Autodesk Fusion 360 part; units mm, degrees
(part 3 of 3)
extrude "돌출9" cut sketch "스케치1" against normal blind 9.6 contours L19 L20 L21 L22 | L23 L24 L25 L26 | L27 L28 L29 L30 bodies 2 in component "leftBody1"
extrude "돌출7'''" add sketch "스케치2 (6)" against normal blind 12 contours L2 L6 L11 L12 L13 L14 L15 L16 L17 L18 | L2 L6 L19 L20 L21 L22 L23 L24 L25 L26 bodies 9 in component "rightPalmRest1"
extrude "돌출8''" cut sketch "스케치2 (6)" against normal blind 12 contours L2 L6 L11 L12 L13 L14 L15 L16 L17 L18 | L2 L6 L19 L20 L21 L22 L23 L24 L25 L26 bodies 9 in component "rightPalmRest1"
extrude "돌출8'''" cut sketch "스케치2 (6)" against normal blind 12 contours L2 L6 L11 L12 L13 L14 L15 L16 L17 L18 | L2 L6 L19 L20 L21 L22 L23 L24 L25 L26 bodies 11 in component "rightPalmRest2"
move_face "면 간격띄우기3" offset -0.5 16 faces at (127.7167, -70, -11) (125.05, -72.6667, -11) (123.05, -74, -11) (122.05, -66, -11) (124.05, -62, -11) (126.3833, -66, -11) (123.05, -67.3333, -3) (122.05, -22, -11) (124.05, -18, -11) (126.3833, -22, -11) (123.05, -23.3333, -3) (127.7167, -26, -11) (125.05, -28.6667, -11) (123.05, -30, -11) (125.05, -64.6667, -11) (125.05, -20.6667, -11) on bodies 11 in component "rightPalmRest2"
extrude "돌출9'" add sketch "스케치2 (6)" against normal blind 12 contours L2 L6 L11 L12 L13 L14 L15 L16 L17 L18 | L2 L6 L19 L20 L21 L22 L23 L24 L25 L26 bodies 9 in component "rightPalmRest1"
component "leftKey1" placed x (1, 0, 0) y (0, 1, 0) z (0, 0, 1) at (0, 0, 0)
component "leftBody1" placed x (1, 0, 0) y (0, 1, 0) z (0, 0, 1) at (0, 0, 0)
component "rightKey1" placed x (1, 0, 0) y (0, 1, 0) z (0, 0, 1) at (0, 0, 0)
component "rightKey2" placed x (1, 0, 0) y (0, 1, 0) z (0, 0, 1) at (0, 0, 0)
component "rightBody1" placed x (1, 0, 0) y (0, 1, 0) z (0, 0, 1) at (0, 0, 0)
component "rightBody2" placed x (1, 0, 0) y (0, 1, 0) z (0, 0, 1) at (0, 0, 0)
component "tempJoin" placed x (1, 0, 0) y (0, 1, 0) z (0, 0, 1) at (13.5824, 154.2275, -3.4182)
component "rightPalmRest1" placed x (1, 0, 0) y (0, 1, 0) z (0, 0, 1) at (0, 0, 0)
component "rightPalmRest2" placed x (1, 0, 0) y (0, 1, 0) z (0, 0, 1) at (0, 0, 0)
component "leftPalmRest2" placed x (1, 0, 0) y (0, 1, 0) z (0, 0, 1) at (0, 0, 0)
component "upper" placed x (1, 0, 0) y (0, 1, 0) z (0, 0, 1) at (0, 0, 0)
equation "keyHoleWidth = 14 mm"
equation "keyWidth = 19.05 mm"
equation "bodyMargin = 4 mm"
equation "boltKeyHole = 3.2 mm"
equation "boltBodyHole = 3 mm"
equation "d6 = boltKeyHole"
equation "bodyBoltCenterMargin = 3.1 mm"
equation "d8 = bodyBoltCenterMargin"
equation "d9 = bodyBoltCenterMargin"
equation "boltHead = 6 mm"
equation "d12 = boltKeyHole"
equation "d14 = bodyBoltCenterMargin"
equation "d15 = bodyBoltCenterMargin"
equation "d16 = ( 1.25 * 4 * keyWidth ) + ( 2.25 * keyWidth ) + bodyMargin * 2"
equation "d17 = ( 5 * keyWidth ) + bodyMargin * 2"
equation "d18 = keyHoleWidth"
equation "d19 = keyHoleWidth"
equation "keyMargin = ( keyWidth - keyHoleWidth ) / 2"
equation "d21 = ( keyWidth * 1.25 - keyHoleWidth ) / 2 + bodyMargin"
equation "d22 = bodyMargin + keyMargin"
equation "d25 = keyWidth * 1.25"
equation "d32 = keyHoleWidth"
equation "d33 = keyHoleWidth"
equation "d37 = keyWidth"
equation "d39 = keyHoleWidth"
equation "d40 = keyHoleWidth"
equation "d41 = ( keyWidth * 1.75 - keyHoleWidth ) / 2 + bodyMargin"
equation "d43 = keyHoleWidth"
equation "d44 = keyHoleWidth"
equation "d45 = ( keyWidth * 1.75 - keyHoleWidth ) / 2 + keyMargin"
equation "d48 = keyWidth"
equation "d50 = keyHoleWidth"
equation "d51 = keyHoleWidth"
equation "d52 = ( keyWidth * 1.5 - keyHoleWidth ) / 2 + bodyMargin"
equation "d53 = keyWidth"
equation "d54 = keyHoleWidth"
equation "d55 = keyHoleWidth"
equation "d56 = ( keyWidth * 1.5 - keyHoleWidth ) / 2 + keyMargin"
equation "d59 = keyWidth"
equation "d61 = keyHoleWidth"
equation "d62 = keyHoleWidth"
equation "d64 = keyMargin + bodyMargin"
equation "d68 = keyWidth"
equation "d70 = keyWidth"
equation "d71 = boltKeyHole"
equation "d73 = bodyBoltCenterMargin"
equation "d74 = boltKeyHole"
equation "d82 = width"
equation "d83 = width"
equation "d85 = stabilHeight"
equation "d87 = ( stabilHeight - 2.2 mm ) / 2"
equation "d88 = ( keyHoleWidth - 2.2 mm ) / 2"
equation "d89 = ( keyWidth * 1.25 - keyHoleWidth ) / 2 + ( keyWidth * 2.25 - keyHoleWidth ) / 2"
equation "d90 = width"
equation "d91 = width"
equation "d93 = stabilHeight"
equation "d95 = ( stabilHeight - 2.2 mm ) / 2"
equation "d96 = ( keyHoleWidth - 2.2 mm ) / 2"
equation "d97 = keyWidth"
equation "d98 = ( keyWidth * 2.25 - keyHoleWidth ) / 2 + bodyMargin"
equation "d99 = keyWidth"
equation "d100 = ( keyWidth * 2.25 - keyHoleWidth ) / 2 + keyMargin"
equation "d101 = keyPlateHeight"
equation "d103 = boltHead"
equation "d104 = boltHead"
equation "d105 = boltHead"
equation "d106 = boltHead"
equation "d107 = -boltHeadDepth"
equation "boltHeadDepth = 1.75 mm"
equation "d136 = ( 1.25 * 4 * keyWidth ) + ( 2.25 * keyWidth ) + bodyMargin * 2"
equation "d137 = boltBodyHole"
equation "d138 = boltBodyHole"
equation "d139 = boltBodyHole"
equation "d140 = bodyBoltCenterMargin"
equation "d141 = boltBodyHole"
equation "d142 = bodyBoltMargin"
equation "bodyBoltMargin = 4.75 mm"
equation "bodyWallDepth = 2.5 mm"
equation "d145 = bodyBoltMargin"
equation "d146 = bodyBoltMargin"
equation "d147 = bodyBoltMargin"
equation "d151 = bodyWallDepth"
equation "d152 = bodyWallDepth"
equation "bodyHeight = 15 mm"
equation "bodyDepth = bodyHeight - 2 mm"
equation "d156 = -bodyHeight"
equation "d158 = -bodyDepth"
equation "bodyBoltHoleDepth = bodyDepth - 3 mm"
equation "d161 = -bodyBoltHoleDepth"
equation "roundRadios = 3.1 mm"
equation "d217 = roundRadios"
equation "keyPlateHeight = 3 mm"
equation "d222 = roundRadios"
equation "d242 = ( ( 18 - ( 5.8 ) ) / 2 ) * 1 mm"
equation "d245 = -bodyWallDepth"
equation "d247 = -bodyWallDepth + 1 mm"
equation "d386 = keyWidth * 5 + bodyMargin * 2"
equation "d392 = width"
equation "d393 = width"
equation "d395 = stabilHeight"
equation "d397 = ( stabilHeight - 2.2 mm ) / 2"
equation "d398 = ( keyHoleWidth - 2.2 mm ) / 2"
equation "d400 = keyHoleWidth"
equation "d401 = keyHoleWidth"
equation "d402 = ( keyWidth * 2.75 - keyHoleWidth ) / 2 + keyMargin"
equation "d443 = boltKeyHole"
equation "d448 = boltKeyHole"
equation "d449 = bodyBoltCenterMargin"
equation "d450 = boltKeyHole"
equation "d451 = bodyBoltCenterMargin"
equation "d491 = keyHoleWidth"
equation "d492 = keyHoleWidth"
equation "d493 = keyMargin + keyWidth + bodyMargin"
equation "d494 = keyMargin + bodyMargin"
equation "d506 = keyHoleWidth"
equation "d507 = keyHoleWidth"
equation "d508 = keyWidth"
equation "d509 = keyHoleWidth"
equation "d510 = keyHoleWidth"
equation "d511 = ( keyWidth * 1.75 - keyHoleWidth ) / 2 + keyMargin"
equation "d512 = keyHoleWidth"
equation "d513 = keyHoleWidth"
equation "d514 = ( keyWidth * 1.75 - keyHoleWidth ) / 2 + keyMargin"
equation "d515 = width"
equation "d516 = width"
equation "d518 = stabilHeight"
equation "d520 = ( stabilHeight - 2.2 mm ) / 2"
equation "d521 = ( keyHoleWidth - 2.2 mm ) / 2"
equation "d522 = keyWidth"
equation "d523 = ( keyWidth * 2.25 - keyHoleWidth ) / 2 + keyWidth + bodyMargin"
equation "d524 = keyHoleWidth"
equation "d525 = keyHoleWidth"
equation "d526 = ( keyWidth * 2.25 - keyHoleWidth ) / 2 + keyMargin"
equation "d527 = keyHoleWidth"
equation "d528 = keyHoleWidth"
equation "d529 = keyWidth"
equation "d530 = ( keyWidth * 1.5 - keyHoleWidth ) / 2 + keyWidth + bodyMargin"
equation "d531 = keyHoleWidth"
equation "d532 = keyHoleWidth"
equation "d533 = ( keyWidth * 1.5 - keyHoleWidth ) / 2 + keyMargin"
equation "d534 = width"
equation "d535 = width"
equation "d537 = stabilHeight"
equation "d539 = ( stabilHeight - 2.2 mm ) / 2"
equation "d540 = ( keyHoleWidth - 2.2 mm ) / 2"
equation "d541 = keyWidth"
equation "d542 = ( keyWidth * 2 - keyHoleWidth ) / 2 + keyWidth + bodyMargin"
equation "d543 = keyHoleWidth"
equation "d544 = keyHoleWidth"
equation "d545 = ( keyWidth * 2 - keyHoleWidth ) / 2 + keyMargin"
equation "d546 = boltKeyHole"
equation "d547 = bodyBoltCenterMargin"
equation "d548 = bodyBoltCenterMargin"
equation "d549 = boltKeyHole"
equation "d550 = bodyBoltCenterMargin"
equation "d555 = keyHoleWidth"
equation "d556 = keyHoleWidth"
equation "d557 = keyMargin + bodyMargin"
equation "d570 = keyHoleWidth"
equation "d571 = keyHoleWidth"
equation "d573 = keyWidth"
equation "d574 = keyWidth"
equation "d575 = keyWidth"
equation "d579 = keyHoleWidth"
equation "d580 = keyHoleWidth"
equation "d581 = keyHoleWidth"
equation "d582 = keyHoleWidth"
equation "d583 = keyHoleWidth"
equation "d584 = keyHoleWidth"
equation "d587 = keyWidth"
equation "d591 = keyWidth"
equation "d595 = keyWidth"
equation "d599 = keyWidth"
equation "d604 = bodyBoltCenterMargin"
equation "d605 = boltKeyHole"
equation "d606 = bodyBoltCenterMargin"
equation "d607 = bodyBoltCenterMargin"
equation "d608 = boltKeyHole"
equation "d609 = bodyBoltCenterMargin"
equation "d610 = bodyBoltCenterMargin"
equation "d614 = boltHead"
equation "d615 = boltHead"
equation "d616 = boltHead"
equation "d617 = boltHead"
equation "d618 = -boltHeadDepth"
equation "d621 = roundRadios"
equation "d622 = bodyMargin * 2 + ( keyWidth * 8 ) + keyWidth * 2 + 30 mm"
equation "d625 = boltKeyHole"
equation "d626 = bodyBoltCenterMargin"
equation "d627 = boltKeyHole"
equation "d628 = boltKeyHole"
equation "d629 = bodyBoltCenterMargin"
equation "d630 = bodyBoltCenterMargin"
equation "d631 = boltKeyHole"
equation "d632 = boltKeyHole"
equation "d633 = boltKeyHole"
equation "d634 = bodyBoltCenterMargin"
equation "d637 = bodyBoltCenterMargin"
equation "d639 = keyPlateHeight"
equation "d641 = boltHead"
equation "d642 = boltHead"
equation "d643 = boltHead"
equation "d644 = boltHead"
equation "d645 = boltHead"
equation "d646 = boltHead"
equation "d647 = boltHead"
equation "d649 = boltHead"
equation "d650 = -boltHeadDepth"
equation "d653 = roundRadios"
equation "d654 = keyPlateHeight"
equation "d656 = boltHead"
equation "d657 = boltHead"
equation "d658 = boltHead"
equation "d659 = boltHead"
equation "d660 = -boltHeadDepth"
equation "d663 = roundRadios"
equation "d664 = boltBodyHole"
equation "d665 = boltBodyHole"
equation "d666 = boltBodyHole"
equation "d667 = boltBodyHole"
equation "d668 = boltBodyHole"
equation "d669 = boltBodyHole"
equation "d670 = boltBodyHole"
equation "d671 = boltBodyHole"
equation "d672 = bodyBoltMargin"
equation "d674 = bodyBoltMargin"
equation "d675 = bodyBoltMargin"
equation "d676 = bodyBoltMargin"
equation "d677 = bodyBoltMargin"
equation "d678 = bodyBoltMargin"
equation "d679 = bodyBoltMargin"
equation "d680 = bodyWallDepth"
equation "d682 = bodyWallDepth"
equation "d683 = bodyWallDepth"
equation "d686 = bodyBoltMargin"
equation "d687 = bodyWallDepth"
equation "d688 = bodyWallDepth"
equation "d689 = bodyWallDepth"
equation "d690 = bodyWallDepth"
equation "d691 = -bodyHeight"
equation "d693 = -bodyDepth"
equation "d695 = -bodyBoltHoleDepth"
equation "d699 = boltBodyHole"
equation "d700 = boltBodyHole"
equation "d701 = boltBodyHole"
equation "d702 = boltBodyHole"
equation "d703 = bodyBoltMargin"
equation "d704 = bodyBoltMargin"
equation "d705 = bodyBoltMargin"
equation "d706 = bodyBoltMargin"
equation "d707 = bodyWallDepth"
equation "d708 = bodyWallDepth"
equation "d710 = bodyWallDepth"
equation "d711 = bodyWallDepth"
equation "d712 = -bodyHeight"
equation "d714 = -bodyDepth"
equation "d716 = -bodyBoltHoleDepth"
equation "d735 = ( 3.6 / 2 ) * 1 mm"
equation "d739 = -bodyWallDepth"
equation "d741 = -bodyWallDepth + 1 mm"
equation "d743 = bodyBoltMargin"
equation "d744 = boltBodyHole"
equation "d745 = boltBodyHole"
equation "d749 = roundRadios"
equation "d751 = roundRadios"
equation "d753 = bodyDepth"
equation "stabilHeight = 11.2 mm"
equation "d767 = bodyDepth"
equation "d773 = bodyDepth"
equation "d777 = palmRestHeight"
equation "d854 = ( 1.25 * 4 * keyWidth ) + ( 2.25 * keyWidth ) + bodyMargin * 2"
equation "d918 = bodyWallDepth"
equation "d919 = bodyWallDepth"
equation "d920 = bodyWallDepth"
equation "magnetThin = 1.2 mm"
equation "magnetWidth = 4.2 mm"
equation "magnetHoleHeight = bodyHeight / 2 + magnetWidth / 2"
equation "d942 = magnetWidth"
equation "d943 = magnetThin"
equation "d950 = -magnetHoleHeight"
equation "palmRestHeight = 20 mm"
